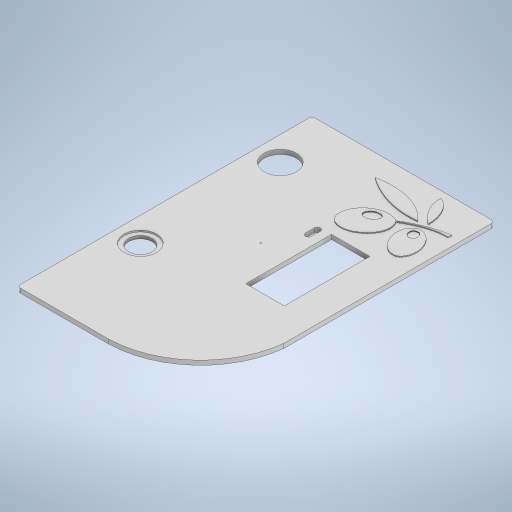
# Autodesk Inventor part: EvoTest_body
Saved by Autodesk Inventor 2023.2 (Build 272271000, 271)
## iProperties
Created: 2022-12-05
Part Number: EvoTest_body
Material: Generico
Document SubType Name: Modeling
Designer: Silvio Marano
Density: 1 g/cm^3
Appearance: Default
Engineer: Silvio Marano
Author: Silvio Marano
Title: EVOTest
Autodesk Inventor part; units mm, degrees
ref_plane "YZ Plane" through (0, 0, 0) normal (1, 0, 0) x (0, 1, 0)
ref_plane "XZ Plane" through (0, 0, 0) normal (0, 1, 0) x (-1, 0, 0)
ref_plane "XY Plane" through (0, 0, 0) normal (0, 0, 1) x (1, 0, 0)
sketch "MainSketch" plane through (0, 0, 0) normal (0, 1, 0) x (-1, 0, 0)
  line L0 (31, -50) -> (-31, -50)
  line L1 (-31, -50) -> (-31, 50)
  line L2 (-31, 50) -> (31, 50)
  line L3 (31, 50) -> (31, -50)
  line L4 (31, -49.4494) -> (-31, 50.5506) construction
  line L5 (-31, -50) -> (31, 50) construction
  line L6 (31, 50) -> (-31, 50)
  line L7 (-31, 50) -> (-31, 21.5)
  line L8 (-31, 21.5) -> (31, 21.5)
  line L9 (31, 21.5) -> (31, 50)
  line L10 (-31, -50) -> (16, -50)
  line L11 (16, -50) -> (16, 21.5)
  line L12 (16, 21.5) -> (-31, 21.5)
  line L13 (-31, 21.5) -> (-31, -50)
  line L14 (31, 21.5) -> (16, 21.5)
  line L15 (16, 21.5) -> (16, -50)
  line L16 (16, -50) -> (31, -50)
  line L17 (31, -50) -> (31, 21.5)
  line L18 (-31, 21.5) -> (-31, 35.75)
  line L19 (-31, 21.5) -> (-31, 35.75)
  arc A0 (0, 50) -> (-31, 21.5) centre (0.8091, 18.0102) ccw
  line L20 (29.5, 48.5) -> (-29.5, 48.5)
  line L21 (-29.5, 48.5) -> (-29.5, -48.5)
  line L22 (-29.5, -48.5) -> (29.5, -48.5)
  line L23 (29.5, -48.5) -> (29.5, 48.5)
  line L24 (29.5, 48.5) -> (-29.5, -48.5) construction
  line L25 (-29.5, 48.5) -> (29.5, -48.5) construction
  line L26 (-29.5, -48.5) -> (16, -48.5)
  line L27 (16, -48.5) -> (16, 2.2597)
  line L28 (16, 2.2597) -> (-29.5, 2.2597)
  line L29 (-29.5, 2.2597) -> (-29.5, -48.5)
  line L30 (16, -48.5) -> (29.5, -48.5)
  line L31 (29.5, -48.5) -> (29.5, 11.5)
  line L32 (29.5, 11.5) -> (16, 11.5)
  line L33 (16, 11.5) -> (16, -48.5)
  line L34 (29.5, 21.5) -> (16, 21.5)
  line L35 (16, 21.5) -> (16, 11.5)
  line L36 (16, 11.5) -> (29.5, 11.5)
  line L37 (29.5, 11.5) -> (29.5, 21.5)
  line L38 (29.5, 21.5) -> (29.5, 11.5)
  line L39 (29.5, 16.5) -> (16, 16.5)
  line L40 (22.75, 16.5) -> (22.75, 11.5)
  line L41 (22.75, 16.5) -> (22.75, 21.5)
  circle A1 centre (22.75, 16.5) radius 4
  arc A2 (0, 48.5) -> (-29.5, 21.5) centre (0.9166, 17.8828) ccw
  line L42 (-20.0675, 15.4609) -> (-7.0675, 15.4609)
  line L43 (-7.0675, 15.4609) -> (-7.0675, -23.5689)
  line L44 (-7.0675, -23.5689) -> (-20.0675, -23.5689)
  line L45 (-20.0675, -23.5689) -> (-20.0675, 15.4609)
  line L46 (22.75, 11.5) -> (22.75, -28.5)
  line L47 (22.75, 11.5) -> (62.75, 11.5) construction
  line L48 (20.2505, -33.5) -> (20.2505, -28.5)
  line L49 (22.75, -28.5) -> (25.2505, -28.5)
  line L50 (20.2505, -28.5) -> (25.2505, -28.5)
  line L51 (25.2505, -28.5) -> (25.2505, -33.5)
  line L52 (25.2505, -33.5) -> (20.2505, -33.5)
  line L53 (20.2505, -33.5) -> (20.2505, -28.5)
  line L54 (25.2505, -28.5) -> (20.2505, -33.5)
  line L55 (20.2505, -28.5) -> (25.2505, -33.5)
  circle A3 centre (22.7505, -31) radius 5.5
  line L56 (-7.0675, 15.4609) -> (-20.0675, 15.4609)
  line L57 (-20.0675, 15.4609) -> (-20.0675, 10.4609)
  line L58 (-20.0675, 10.4609) -> (-7.0675, 10.4609)
  line L59 (-7.0675, 10.4609) -> (-7.0675, 15.4609)
  line L60 (-7.0675, -23.5689) -> (-20.0675, -23.5689)
  line L61 (-20.0675, -23.5689) -> (-20.0675, -18.5689)
  line L62 (-20.0675, -18.5689) -> (-7.0675, -18.5689)
  line L63 (-7.0675, -18.5689) -> (-7.0675, -23.5689)
  line L64 (-29.5, -48.5) -> (-16.5, -48.5)
  line L65 (-16.5, -48.5) -> (-8.5, -48.5)
  line L66 (-8.5, -48.5) -> (-8.5, -42.5)
  line L67 (-8.5, -42.5) -> (-16.5, -42.5)
  line L68 (-16.5, -42.5) -> (-16.5, -48.5)
  line L69 (-8.5, -42.5) -> (-4.5, -42.5)
  line L70 (-8.5, -42.5) -> (-4.5, -42.5) construction
  line L71 (-4.5, -42.5) -> (-3.5, -42.5)
  line L72 (-3.5, -42.5) -> (-3.5, -40.5)
  line L73 (-3.5, -40.5) -> (-4.5, -40.5)
  line L74 (-4.5, -40.5) -> (-4.5, -42.5)
  line L75 (-4.5, -42.5) -> (-3.5, -42.5)
  line L76 (-3.5, -42.5) -> (-3.5, -44.5)
  line L77 (-3.5, -44.5) -> (-4.5, -44.5)
  line L78 (-4.5, -44.5) -> (-4.5, -42.5)
  line L79 (-8.5, -42.5) -> (-8.5, -10.5)
  line L80 (-8.5, -10.5) -> (-10.5, -10.5)
  line L81 (-10.5, -10.5) -> (-10.5, -9.5)
  line L82 (-10.5, -9.5) -> (-8.5, -9.5)
  line L83 (-8.5, -9.5) -> (-8.5, -10.5)
  line L84 (-8.5, -42.5) -> (-8.5, -37.5)
  line L85 (-8.5, -37.5) -> (-9.5, -37.5)
  line L86 (-9.5, -37.5) -> (-9.5, -39.5)
  line L87 (-9.5, -39.5) -> (-8.5, -39.5)
  line L88 (-8.5, -39.5) -> (-8.5, -37.5)
  point P0 (0, 0)
  dimension "d0" = 62
  dimension "d1" = 100
  dimension "d2" = 62
  dimension "d3" = 28.5
  dimension "d4" = 47
  dimension "d5" = 32
  dimension "d6" = 59
  dimension "d7" = 97
  dimension "d8" = 60
  dimension "d9" = 8
  dimension "d10" = 39.0299
  dimension "d11" = 13
  dimension "d12" = 40
  dimension "d13" = 90
  dimension "d14" = 5
  dimension "d15" = 5
  dimension "d16" = 11
  dimension "d17" = 5
  dimension "d18" = 5
  dimension "d19" = 13
  dimension "d20" = 8
  dimension "d21" = 6
  dimension "d22" = 4
  dimension "d23" = 0
  dimension "d24" = 1
  dimension "d25" = 2
  dimension "d26" = 2
  dimension "d27" = 32
  dimension "d28" = 2
  dimension "d29" = 1
  dimension "d30" = 5
  dimension "d31" = 1
  dimension "d32" = 2
  constraints: 178 end point, 32 parallel, 21 perpendicular, 19 horizontal, 12 midpoint, 12 point on line, 4 centre point, 4 point on circle, 2 equal length, 2 vertical, 1 coincident, 1 collinear
  measures "d0" distance of L2.start L2.end
  measures "d1" distance of L3.end L2.end
  measures "d2" distance of L8.end L7.end
  measures "d3" distance of L7.end L6.end
  measures "d4" distance of L12.end L11.end
  measures "d5" radius of A0
  measures "d6" distance of L22.end L21.end
  measures "d7" distance of L21.end L20.end
  measures "d8" distance of L31.end L30.end
  measures "d9" diameter of A1
  measures "d10" distance of L44.end L42.start
  measures "d11" distance of L43.end L44.end
  measures "d12" distance of L40.end L46.end
  measures "d13" angle of L46 L47
  measures "d14" distance of L51.end L48.start
  measures "d15" distance of L49.end L51.end
  measures "d16" diameter of A3
  measures "d17" distance of L57.end L56.end
  measures "d18" distance of L60.end L61.end
  measures "d19" distance of L21.end L64.end
  measures "d20" distance of L67.end L66.end
  measures "d21" distance of L66.end L65.end
  measures "d22" distance of L66.end L69.end
  measures "d23" distance between parallel lines of L69 L70
  measures "d24" distance of L73.end L72.end
  measures "d25" distance of L72.end L71.end
  measures "d26" distance of L75.end L76.end
  measures "d27" distance of L66.end L79.end
  measures "d28" distance of L79.end L80.end
  measures "d29" distance of L80.end L81.end
  measures "d30" distance of L66.end L84.end
  measures "d31" distance of L87.end L86.end
  measures "d32" distance of L86.end L85.end
extrude "MainExtrusion" add sketch "MainSketch" along normal blind 1.5 contours L0 L11 L22 L23 L8 L3 | L0 L1 L8 L21 L22 L11 | L8 L23 L20 A0 L2 L3 | L22 L66 L79 L44 L43 L28 L11 | L11 L32 L23 L22 | L23 L39 A1 L41 L8 | L8 A2 L20 L23 | A0 L21 L8 | L28 L43 L42 L45 L21 L8 L11 | L22 L68 L67 L66 | L41 A1 L39 L11 L8 | L23 L32 L40 A1 L39 | L21 A0 L20 A2 | L11 L39 A1 L40 L32 | L22 L21 L28 L45 L44 L79 L85 L86 L87 L67 L68 | L58 L45 L42 L43 | L43 L44 L79 L62 | L87 L86 L85 L79 | L62 L79 L44 L45 | L74 L73 L72 L71 | L71 L76 L77 L78
sketch "LedSketch" plane through (0, 1.5, 0) normal (0, 1, 0) x (1, 0, 0)
  line L0 (4.2664, 18.5689) -> (2.2664, 18.5689)
  line L1 (2.2664, 18.5689) -> (2.2664, 13.5689)
  line L2 (2.2664, 13.5689) -> (4.2664, 13.5689)
  line L3 (4.2664, 13.5689) -> (4.2664, 18.5689)
  point P0 (0, 0)
  dimension "d35" = 2
  dimension "d36" = 5
  constraints: 8 end point, 2 parallel, 1 horizontal, 1 perpendicular
  measures "d35" distance of L2.end L1.end
  measures "d36" distance of L1.end L0.end
extrude "LedCutExtrusion" cut sketch "LedSketch" against normal blind 1.5
fillet "EdgeConnection" radius 1 3 edges at (-31, 0.75, 50) (-31, 0.75, -50) (31, 0.75, -50)
fillet "LedConnection" radius 1 4 edges at (2.2664, 0.75, -18.5689) (4.2664, 0.75, -18.5689) (4.2664, 0.75, -13.5689) (2.2664, 0.75, -13.5689)
sketch "PipetePlacementSketch" plane through (0, 1.5, 0) normal (0, 1, 0) x (1, 0, 0)
  circle A0 centre (-22.7505, 31) radius 5.5 projected
  line L0 (-17.2505, 31) -> (-17.2505, -16.8177)
  line L1 (-28.2505, 31) -> (-28.2505, -16.8177)
  circle A1 centre (-22.75, -16.5) radius 4 projected
  circle A2 centre (-22.75, -16.5) radius 5.5
  point P0 (0, 0)
  dimension "d41" = 11
  constraints: 4 end point, 2 point on circle, 2 vertical, 1 centre point, 1 coincident, 1 tangent
  measures "d41" diameter of A2
extrude "PipettePlacementExtrusion" cut sketch "PipetePlacementSketch" against normal blind 0.5 contours A2 | A1
sketch "OliveSketch" plane through (0, 1.5, 0) normal (0, 1, 0) x (1, 0, 0)
  line L0 (15.3803, 47.4947) -> (15.7568, 47.3174)
  line L1 (15.7568, 47.3174) -> (16.1189, 47.1219)
  line L2 (16.1189, 47.1219) -> (16.4667, 46.9087)
  line L3 (16.4667, 46.9087) -> (16.8002, 46.6788)
  line L4 (16.8002, 46.6788) -> (17.1196, 46.4328)
  line L5 (17.1196, 46.4328) -> (17.4248, 46.1716)
  line L6 (17.4248, 46.1716) -> (17.716, 45.896)
  line L7 (17.716, 45.896) -> (17.9932, 45.6067)
  line L8 (17.9932, 45.6067) -> (18.2565, 45.3044)
  line L9 (18.2565, 45.3044) -> (18.5059, 44.99)
  line L10 (18.5059, 44.99) -> (18.7416, 44.6642)
  line L11 (18.7416, 44.6642) -> (18.9635, 44.3278)
  line L12 (18.9635, 44.3278) -> (19.1717, 43.9816)
  line L13 (19.1717, 43.9816) -> (19.3664, 43.6263)
  line L14 (19.3664, 43.6263) -> (19.5475, 43.2628)
  line L15 (19.5475, 43.2628) -> (19.7151, 42.8917)
  line L16 (19.7151, 42.8917) -> (19.8694, 42.5139)
  line L17 (19.8694, 42.5139) -> (20.0103, 42.1301)
  line L18 (20.0103, 42.1301) -> (20.138, 41.7412)
  line L19 (20.138, 41.7412) -> (20.2525, 41.3478)
  line L20 (20.2525, 41.3478) -> (20.3538, 40.9508)
  line L21 (20.3538, 40.9508) -> (20.4421, 40.5509)
  line L22 (20.4421, 40.5509) -> (20.5173, 40.1489)
  line L23 (20.5173, 40.1489) -> (20.5796, 39.7455)
  line L24 (20.5796, 39.7455) -> (20.6291, 39.3416)
  line L25 (20.6291, 39.3416) -> (20.6657, 38.938)
  line L26 (20.6657, 38.938) -> (20.6896, 38.5353)
  line L27 (20.6896, 38.5353) -> (20.7009, 38.1344)
  line L28 (20.7009, 38.1344) -> (20.6995, 37.736)
  line L29 (20.6995, 37.736) -> (20.377, 37.9653)
  line L30 (20.377, 37.9653) -> (20.0601, 38.2051)
  line L31 (20.0601, 38.2051) -> (19.7493, 38.4548)
  line L32 (19.7493, 38.4548) -> (19.4452, 38.7144)
  line L33 (19.4452, 38.7144) -> (19.1481, 38.9834)
  line L34 (19.1481, 38.9834) -> (18.8586, 39.2615)
  line L35 (18.8586, 39.2615) -> (18.5771, 39.5486)
  line L36 (18.5771, 39.5486) -> (18.3041, 39.8442)
  line L37 (18.3041, 39.8442) -> (18.04, 40.148)
  line L38 (18.04, 40.148) -> (17.7855, 40.4598)
  line L39 (17.7855, 40.4598) -> (17.5409, 40.7792)
  line L40 (17.5409, 40.7792) -> (17.3067, 41.106)
  line L41 (17.3067, 41.106) -> (17.0833, 41.4399)
  line L42 (17.0833, 41.4399) -> (16.8714, 41.7805)
  line L43 (16.8714, 41.7805) -> (16.6713, 42.1275)
  line L44 (16.6713, 42.1275) -> (16.4835, 42.4807)
  line L45 (16.4835, 42.4807) -> (16.3085, 42.8398)
  line L46 (16.3085, 42.8398) -> (16.1468, 43.2044)
  line L47 (16.1468, 43.2044) -> (15.9988, 43.5742)
  line L48 (15.9988, 43.5742) -> (15.8651, 43.949)
  line L49 (15.8651, 43.949) -> (15.746, 44.3284)
  line L50 (15.746, 44.3284) -> (15.6422, 44.7121)
  line L51 (15.6422, 44.7121) -> (15.554, 45.0999)
  line L52 (15.554, 45.0999) -> (15.4819, 45.4915)
  line L53 (15.4819, 45.4915) -> (15.4265, 45.8865)
  line L54 (15.4265, 45.8865) -> (15.3881, 46.2846)
  line L55 (15.3881, 46.2846) -> (15.3673, 46.6855)
  line L56 (15.3673, 46.6855) -> (15.3646, 47.089)
  line L57 (15.3646, 47.089) -> (15.3803, 47.4947)
  line L58 (-1.9352, 42.3819) -> (-1.212, 42.5249)
  line L59 (-1.212, 42.5249) -> (-0.4813, 42.6475)
  line L60 (-0.4813, 42.6475) -> (0.2559, 42.7493)
  line L61 (0.2559, 42.7493) -> (0.9983, 42.8299)
  line L62 (0.9983, 42.8299) -> (1.7448, 42.889)
  line L63 (1.7448, 42.889) -> (2.4944, 42.9262)
  line L64 (2.4944, 42.9262) -> (3.2458, 42.9412)
  line L65 (3.2458, 42.9412) -> (3.9981, 42.9335)
  line L66 (3.9981, 42.9335) -> (4.75, 42.9028)
  line L67 (4.75, 42.9028) -> (5.5004, 42.8488)
  line L68 (5.5004, 42.8488) -> (6.2482, 42.7711)
  line L69 (6.2482, 42.7711) -> (6.9923, 42.6693)
  line L70 (6.9923, 42.6693) -> (7.7316, 42.543)
  line L71 (7.7316, 42.543) -> (8.4649, 42.3919)
  line L72 (8.4649, 42.3919) -> (9.1912, 42.2157)
  line L73 (9.1912, 42.2157) -> (9.9092, 42.0139)
  line L74 (9.9092, 42.0139) -> (10.6179, 41.7862)
  line L75 (10.6179, 41.7862) -> (11.3162, 41.5323)
  line L76 (11.3162, 41.5323) -> (12.0029, 41.2517)
  line L77 (12.0029, 41.2517) -> (12.6769, 40.9442)
  line L78 (12.6769, 40.9442) -> (13.337, 40.6093)
  line L79 (13.337, 40.6093) -> (13.9823, 40.2466)
  line L80 (13.9823, 40.2466) -> (14.6115, 39.8559)
  line L81 (14.6115, 39.8559) -> (15.2234, 39.4367)
  line L82 (15.2234, 39.4367) -> (15.8171, 38.9888)
  line L83 (15.8171, 38.9888) -> (16.3914, 38.5116)
  line L84 (16.3914, 38.5116) -> (16.9451, 38.0049)
  line L85 (16.9451, 38.0049) -> (17.4771, 37.4683)
  line L86 (17.4771, 37.4683) -> (17.9864, 36.9015)
  line L87 (17.9864, 36.9015) -> (17.2597, 36.8206)
  line L88 (17.2597, 36.8206) -> (16.5319, 36.7617)
  line L89 (16.5319, 36.7617) -> (15.8036, 36.7245)
  line L90 (15.8036, 36.7245) -> (15.0751, 36.7088)
  line L91 (15.0751, 36.7088) -> (14.3468, 36.7142)
  line L92 (14.3468, 36.7142) -> (13.6192, 36.7403)
  line L93 (13.6192, 36.7403) -> (12.8927, 36.787)
  line L94 (12.8927, 36.787) -> (12.1677, 36.8539)
  line L95 (12.1677, 36.8539) -> (11.4447, 36.9407)
  line L96 (11.4447, 36.9407) -> (10.7242, 37.0471)
  line L97 (10.7242, 37.0471) -> (10.0064, 37.1727)
  line L98 (10.0064, 37.1727) -> (9.292, 37.3173)
  line L99 (9.292, 37.3173) -> (8.5812, 37.4806)
  line L100 (8.5812, 37.4806) -> (7.8746, 37.6623)
  line L101 (7.8746, 37.6623) -> (7.1725, 37.862)
  line L102 (7.1725, 37.862) -> (6.4755, 38.0794)
  line L103 (6.4755, 38.0794) -> (5.7838, 38.3143)
  line L104 (5.7838, 38.3143) -> (5.098, 38.5663)
  line L105 (5.098, 38.5663) -> (4.4186, 38.8352)
  line L106 (4.4186, 38.8352) -> (3.7458, 39.1205)
  line L107 (3.7458, 39.1205) -> (3.0802, 39.4221)
  line L108 (3.0802, 39.4221) -> (2.4222, 39.7396)
  line L109 (2.4222, 39.7396) -> (1.7722, 40.0727)
  line L110 (1.7722, 40.0727) -> (1.1306, 40.4211)
  line L111 (1.1306, 40.4211) -> (0.498, 40.7845)
  line L112 (0.498, 40.7845) -> (-0.1254, 41.1626)
  line L113 (-0.1254, 41.1626) -> (-0.739, 41.555)
  line L114 (-0.739, 41.555) -> (-1.3424, 41.9616)
  line L115 (-1.3424, 41.9616) -> (-1.9352, 42.3819)
  line L116 (14.2641, 33.2049) -> (14.7001, 33.4684)
  line L117 (14.7001, 33.4684) -> (15.1391, 33.7274)
  line L118 (15.1391, 33.7274) -> (15.5812, 33.9817)
  line L119 (15.5812, 33.9817) -> (16.0262, 34.2311)
  line L120 (16.0262, 34.2311) -> (16.4741, 34.4756)
  line L121 (16.4741, 34.4756) -> (16.925, 34.7148)
  line L122 (16.925, 34.7148) -> (17.3787, 34.9488)
  line L123 (17.3787, 34.9488) -> (17.8352, 35.1773)
  line L124 (17.8352, 35.1773) -> (18.2944, 35.4002)
  line L125 (18.2944, 35.4002) -> (18.7564, 35.6173)
  line L126 (18.7564, 35.6173) -> (19.221, 35.8285)
  line L127 (19.221, 35.8285) -> (19.6883, 36.0335)
  line L128 (19.6883, 36.0335) -> (20.1582, 36.2324)
  line L129 (20.1582, 36.2324) -> (20.6306, 36.4248)
  line L130 (20.6306, 36.4248) -> (21.1055, 36.6107)
  line L131 (21.1055, 36.6107) -> (21.5829, 36.7898)
  line L132 (21.5829, 36.7898) -> (22.0627, 36.9621)
  line L133 (22.0627, 36.9621) -> (22.5449, 37.1273)
  line L134 (22.5449, 37.1273) -> (23.0294, 37.2854)
  line L135 (23.0294, 37.2854) -> (23.5162, 37.436)
  line L136 (23.5162, 37.436) -> (24.0052, 37.5792)
  line L137 (24.0052, 37.5792) -> (24.4965, 37.7147)
  line L138 (24.4965, 37.7147) -> (24.9899, 37.8424)
  line L139 (24.9899, 37.8424) -> (25.4855, 37.9621)
  line L140 (25.4855, 37.9621) -> (25.9831, 38.0736)
  line L141 (25.9831, 38.0736) -> (26.4828, 38.1769)
  line L142 (26.4828, 38.1769) -> (26.9845, 38.2717)
  line L143 (26.9845, 38.2717) -> (27.4882, 38.3579)
  line L144 (27.4882, 38.3579) -> (27.9937, 38.4353)
  line L145 (27.9937, 38.4353) -> (27.8198, 37.2908)
  line L146 (27.8198, 37.2908) -> (27.3273, 37.294)
  line L147 (27.3273, 37.294) -> (26.8366, 37.2826)
  line L148 (26.8366, 37.2826) -> (26.3475, 37.2569)
  line L149 (26.3475, 37.2569) -> (25.8603, 37.2173)
  line L150 (25.8603, 37.2173) -> (25.375, 37.1643)
  line L151 (25.375, 37.1643) -> (24.8916, 37.0983)
  line L152 (24.8916, 37.0983) -> (24.4103, 37.0197)
  line L153 (24.4103, 37.0197) -> (23.9311, 36.9289)
  line L154 (23.9311, 36.9289) -> (23.4541, 36.8264)
  line L155 (23.4541, 36.8264) -> (22.9794, 36.7127)
  line L156 (22.9794, 36.7127) -> (22.5071, 36.5881)
  line L157 (22.5071, 36.5881) -> (22.0372, 36.453)
  line L158 (22.0372, 36.453) -> (21.5697, 36.3079)
  line L159 (21.5697, 36.3079) -> (21.1049, 36.1533)
  line L160 (21.1049, 36.1533) -> (20.6426, 35.9894)
  line L161 (20.6426, 35.9894) -> (20.1832, 35.8169)
  line L162 (20.1832, 35.8169) -> (19.7265, 35.6361)
  line L163 (19.7265, 35.6361) -> (19.2727, 35.4473)
  line L164 (19.2727, 35.4473) -> (18.8218, 35.2512)
  line L165 (18.8218, 35.2512) -> (18.374, 35.048)
  line L166 (18.374, 35.048) -> (17.9292, 34.8382)
  line L167 (17.9292, 34.8382) -> (17.4877, 34.6223)
  line L168 (17.4877, 34.6223) -> (17.0493, 34.4006)
  line L169 (17.0493, 34.4006) -> (16.6143, 34.1737)
  line L170 (16.6143, 34.1737) -> (16.1828, 33.9418)
  line L171 (16.1828, 33.9418) -> (15.7546, 33.7055)
  line L172 (15.7546, 33.7055) -> (15.3301, 33.4652)
  line L173 (15.3301, 33.4652) -> (14.9091, 33.2212)
  line L174 (14.9091, 33.2212) -> (14.4919, 32.9741)
  line L175 (14.4919, 32.9741) -> (14.7249, 32.6067)
  line L176 (14.7249, 32.6067) -> (14.9206, 32.2342)
  line L177 (14.9206, 32.2342) -> (15.0804, 31.8573)
  line L178 (15.0804, 31.8573) -> (15.2055, 31.4771)
  line L179 (15.2055, 31.4771) -> (15.2972, 31.0942)
  line L180 (15.2972, 31.0942) -> (15.3568, 30.7095)
  line L181 (15.3568, 30.7095) -> (15.3855, 30.3239)
  line L182 (15.3855, 30.3239) -> (15.3846, 29.9381)
  line L183 (15.3846, 29.9381) -> (15.3553, 29.5531)
  line L184 (15.3553, 29.5531) -> (15.299, 29.1696)
  line L185 (15.299, 29.1696) -> (15.2169, 28.7884)
  line L186 (15.2169, 28.7884) -> (15.1103, 28.4104)
  line L187 (15.1103, 28.4104) -> (14.9804, 28.0364)
  line L188 (14.9804, 28.0364) -> (14.8285, 27.6673)
  line L189 (14.8285, 27.6673) -> (14.656, 27.3039)
  line L190 (14.656, 27.3039) -> (14.464, 26.9469)
  line L191 (14.464, 26.9469) -> (14.2538, 26.5973)
  line L192 (14.2538, 26.5973) -> (14.0267, 26.2559)
  line L193 (14.0267, 26.2559) -> (13.784, 25.9234)
  line L194 (13.784, 25.9234) -> (13.5269, 25.6008)
  line L195 (13.5269, 25.6008) -> (13.2567, 25.2888)
  line L196 (13.2567, 25.2888) -> (12.9747, 24.9883)
  line L197 (12.9747, 24.9883) -> (12.6821, 24.7001)
  line L198 (12.6821, 24.7001) -> (12.3803, 24.4251)
  line L199 (12.3803, 24.4251) -> (12.0705, 24.164)
  line L200 (12.0705, 24.164) -> (11.7539, 23.9177)
  line L201 (11.7539, 23.9177) -> (11.4318, 23.687)
  line L202 (11.4318, 23.687) -> (11.1056, 23.4728)
  line L203 (11.1056, 23.4728) -> (10.7764, 23.2759)
  line L204 (10.7764, 23.2759) -> (10.5074, 23.1056)
  line L205 (10.5074, 23.1056) -> (10.2247, 22.9458)
  line L206 (10.2247, 22.9458) -> (9.9297, 22.797)
  line L207 (9.9297, 22.797) -> (9.6237, 22.6599)
  line L208 (9.6237, 22.6599) -> (9.3081, 22.5351)
  line L209 (9.3081, 22.5351) -> (8.9843, 22.4231)
  line L210 (8.9843, 22.4231) -> (8.6537, 22.3245)
  line L211 (8.6537, 22.3245) -> (8.3176, 22.2399)
  line L212 (8.3176, 22.2399) -> (7.9775, 22.1699)
  line L213 (7.9775, 22.1699) -> (7.6347, 22.1151)
  line L214 (7.6347, 22.1151) -> (7.2907, 22.076)
  line L215 (7.2907, 22.076) -> (6.9467, 22.0534)
  line L216 (6.9467, 22.0534) -> (6.6042, 22.0476)
  line L217 (6.6042, 22.0476) -> (6.2645, 22.0594)
  line L218 (6.2645, 22.0594) -> (5.9291, 22.0894)
  line L219 (5.9291, 22.0894) -> (5.5993, 22.138)
  line L220 (5.5993, 22.138) -> (5.2765, 22.2059)
  line L221 (5.2765, 22.2059) -> (4.9621, 22.2937)
  line L222 (4.9621, 22.2937) -> (4.6574, 22.402)
  line L223 (4.6574, 22.402) -> (4.3639, 22.5313)
  line L224 (4.3639, 22.5313) -> (4.0829, 22.6823)
  line L225 (4.0829, 22.6823) -> (3.8158, 22.8555)
  line L226 (3.8158, 22.8555) -> (3.564, 23.0515)
  line L227 (3.564, 23.0515) -> (3.3289, 23.271)
  line L228 (3.3289, 23.271) -> (3.1119, 23.5144)
  line L229 (3.1119, 23.5144) -> (2.9142, 23.7824)
  line L230 (2.9142, 23.7824) -> (2.7374, 24.0756)
  line L231 (2.7374, 24.0756) -> (2.5828, 24.3945)
  line L232 (2.5828, 24.3945) -> (2.4518, 24.7398)
  line L233 (2.4518, 24.7398) -> (2.3711, 25.345)
  line L234 (2.3711, 25.345) -> (2.3498, 25.947)
  line L235 (2.3498, 25.947) -> (2.3852, 26.5437)
  line L236 (2.3852, 26.5437) -> (2.4747, 27.133)
  line L237 (2.4747, 27.133) -> (2.6154, 27.7128)
  line L238 (2.6154, 27.7128) -> (2.8045, 28.281)
  line L239 (2.8045, 28.281) -> (3.0395, 28.8353)
  line L240 (3.0395, 28.8353) -> (3.3175, 29.3737)
  line L241 (3.3175, 29.3737) -> (3.6358, 29.894)
  line L242 (3.6358, 29.894) -> (3.9918, 30.394)
  line L243 (3.9918, 30.394) -> (4.3826, 30.8717)
  line L244 (4.3826, 30.8717) -> (4.8055, 31.3249)
  line L245 (4.8055, 31.3249) -> (5.2578, 31.7514)
  line L246 (5.2578, 31.7514) -> (5.7368, 32.1491)
  line L247 (5.7368, 32.1491) -> (6.2398, 32.5159)
  line L248 (6.2398, 32.5159) -> (6.7639, 32.8496)
  line L249 (6.7639, 32.8496) -> (7.3065, 33.1481)
  line L250 (7.3065, 33.1481) -> (7.8649, 33.4092)
  line L251 (7.8649, 33.4092) -> (8.4362, 33.6309)
  line L252 (8.4362, 33.6309) -> (9.0178, 33.8109)
  line L253 (9.0178, 33.8109) -> (9.607, 33.9471)
  line L254 (9.607, 33.9471) -> (10.201, 34.0375)
  line L255 (10.201, 34.0375) -> (10.7971, 34.0798)
  line L256 (10.7971, 34.0798) -> (11.3925, 34.072)
  line L257 (11.3925, 34.072) -> (11.9845, 34.0118)
  line L258 (11.9845, 34.0118) -> (12.5704, 33.8971)
  line L259 (12.5704, 33.8971) -> (13.1475, 33.7259)
  line L260 (13.1475, 33.7259) -> (13.713, 33.4958)
  line L261 (13.713, 33.4958) -> (14.2641, 33.2049)
  line L262 (8.4112, 32.4895) -> (8.2751, 32.4544)
  line L263 (8.2751, 32.4544) -> (8.1391, 32.4101)
  line L264 (8.1391, 32.4101) -> (8.0036, 32.3573)
  line L265 (8.0036, 32.3573) -> (7.8693, 32.2961)
  line L266 (7.8693, 32.2961) -> (7.7369, 32.2272)
  line L267 (7.7369, 32.2272) -> (7.6068, 32.1508)
  line L268 (7.6068, 32.1508) -> (7.4798, 32.0674)
  line L269 (7.4798, 32.0674) -> (7.3563, 31.9773)
  line L270 (7.3563, 31.9773) -> (7.2371, 31.8811)
  line L271 (7.2371, 31.8811) -> (7.1227, 31.7792)
  line L272 (7.1227, 31.7792) -> (7.0137, 31.6718)
  line L273 (7.0137, 31.6718) -> (6.9108, 31.5595)
  line L274 (6.9108, 31.5595) -> (6.8144, 31.4427)
  line L275 (6.8144, 31.4427) -> (6.7253, 31.3217)
  line L276 (6.7253, 31.3217) -> (6.6441, 31.197)
  line L277 (6.6441, 31.197) -> (6.5712, 31.069)
  line L278 (6.5712, 31.069) -> (6.5074, 30.9381)
  line L279 (6.5074, 30.9381) -> (6.4533, 30.8048)
  line L280 (6.4533, 30.8048) -> (6.4094, 30.6693)
  line L281 (6.4094, 30.6693) -> (6.3763, 30.5323)
  line L282 (6.3763, 30.5323) -> (6.3547, 30.3939)
  line L283 (6.3547, 30.3939) -> (6.3451, 30.2548)
  line L284 (6.3451, 30.2548) -> (6.3482, 30.1152)
  line L285 (6.3482, 30.1152) -> (6.3645, 29.9757)
  line L286 (6.3645, 29.9757) -> (6.3947, 29.8365)
  line L287 (6.3947, 29.8365) -> (6.4394, 29.6982)
  line L288 (6.4394, 29.6982) -> (6.4991, 29.5611)
  line L289 (6.4991, 29.5611) -> (6.5745, 29.4257)
  line L290 (6.5745, 29.4257) -> (6.6661, 29.2923)
  line L291 (6.6661, 29.2923) -> (6.8504, 29.1836)
  line L292 (6.8504, 29.1836) -> (7.0433, 29.0952)
  line L293 (7.0433, 29.0952) -> (7.2436, 29.0262)
  line L294 (7.2436, 29.0262) -> (7.4498, 28.9763)
  line L295 (7.4498, 28.9763) -> (7.6608, 28.9447)
  line L296 (7.6608, 28.9447) -> (7.8752, 28.9308)
  line L297 (7.8752, 28.9308) -> (8.0918, 28.9341)
  line L298 (8.0918, 28.9341) -> (8.3092, 28.9539)
  line L299 (8.3092, 28.9539) -> (8.5261, 28.9897)
  line L300 (8.5261, 28.9897) -> (8.7413, 29.0407)
  line L301 (8.7413, 29.0407) -> (8.9535, 29.1065)
  line L302 (8.9535, 29.1065) -> (9.1614, 29.1864)
  line L303 (9.1614, 29.1864) -> (9.3636, 29.2798)
  line L304 (9.3636, 29.2798) -> (9.5589, 29.3861)
  line L305 (9.5589, 29.3861) -> (9.7461, 29.5047)
  line L306 (9.7461, 29.5047) -> (9.9237, 29.635)
  line L307 (9.9237, 29.635) -> (10.0905, 29.7763)
  line L308 (10.0905, 29.7763) -> (10.2452, 29.9282)
  line L309 (10.2452, 29.9282) -> (10.3866, 30.0899)
  line L310 (10.3866, 30.0899) -> (10.5133, 30.2609)
  line L311 (10.5133, 30.2609) -> (10.624, 30.4405)
  line L312 (10.624, 30.4405) -> (10.7175, 30.6282)
  line L313 (10.7175, 30.6282) -> (10.7924, 30.8233)
  line L314 (10.7924, 30.8233) -> (10.8474, 31.0253)
  line L315 (10.8474, 31.0253) -> (10.8814, 31.2335)
  line L316 (10.8814, 31.2335) -> (10.8929, 31.4473)
  line L317 (10.8929, 31.4473) -> (10.8806, 31.6661)
  line L318 (10.8806, 31.6661) -> (10.8434, 31.8894)
  line L319 (10.8434, 31.8894) -> (10.7798, 32.1165)
  line L320 (10.7798, 32.1165) -> (10.7195, 32.1834)
  line L321 (10.7195, 32.1834) -> (10.656, 32.2445)
  line L322 (10.656, 32.2445) -> (10.5896, 32.3001)
  line L323 (10.5896, 32.3001) -> (10.5204, 32.3504)
  line L324 (10.5204, 32.3504) -> (10.4486, 32.3955)
  line L325 (10.4486, 32.3955) -> (10.3744, 32.4358)
  line L326 (10.3744, 32.4358) -> (10.298, 32.4713)
  line L327 (10.298, 32.4713) -> (10.2195, 32.5023)
  line L328 (10.2195, 32.5023) -> (10.1391, 32.5291)
  line L329 (10.1391, 32.5291) -> (10.057, 32.5518)
  line L330 (10.057, 32.5518) -> (9.8884, 32.5858)
  line L331 (9.8884, 32.5858) -> (9.7152, 32.6061)
  line L332 (9.7152, 32.6061) -> (9.4497, 32.6144)
  line L333 (9.4497, 32.6144) -> (9.0927, 32.593)
  line L334 (9.0927, 32.593) -> (8.4112, 32.4895)
  line L335 (20.5124, 34.6997) -> (21.0739, 34.7213)
  line L336 (21.0739, 34.7213) -> (21.6187, 34.6781)
  line L337 (21.6187, 34.6781) -> (22.1456, 34.5739)
  line L338 (22.1456, 34.5739) -> (22.653, 34.4126)
  line L339 (22.653, 34.4126) -> (23.1394, 34.1979)
  line L340 (23.1394, 34.1979) -> (23.6034, 33.9337)
  line L341 (23.6034, 33.9337) -> (24.0436, 33.6239)
  line L342 (24.0436, 33.6239) -> (24.4585, 33.2723)
  line L343 (24.4585, 33.2723) -> (24.8467, 32.8827)
  line L344 (24.8467, 32.8827) -> (25.2066, 32.459)
  line L345 (25.2066, 32.459) -> (25.537, 32.0049)
  line L346 (25.537, 32.0049) -> (25.8362, 31.5244)
  line L347 (25.8362, 31.5244) -> (26.1028, 31.0212)
  line L348 (26.1028, 31.0212) -> (26.3354, 30.4993)
  line L349 (26.3354, 30.4993) -> (26.5326, 29.9623)
  line L350 (26.5326, 29.9623) -> (26.6929, 29.4143)
  line L351 (26.6929, 29.4143) -> (26.8148, 28.8589)
  line L352 (26.8148, 28.8589) -> (26.8968, 28.3001)
  line L353 (26.8968, 28.3001) -> (26.9378, 27.7416)
  line L354 (26.9378, 27.7416) -> (26.9358, 27.1874)
  line L355 (26.9358, 27.1874) -> (26.8897, 26.6412)
  line L356 (26.8897, 26.6412) -> (26.7979, 26.1069)
  line L357 (26.7979, 26.1069) -> (26.659, 25.5883)
  line L358 (26.659, 25.5883) -> (26.4716, 25.0893)
  line L359 (26.4716, 25.0893) -> (26.2343, 24.6137)
  line L360 (26.2343, 24.6137) -> (25.9454, 24.1653)
  line L361 (25.9454, 24.1653) -> (25.6037, 23.7479)
  line L362 (25.6037, 23.7479) -> (25.2077, 23.3655)
  line L363 (25.2077, 23.3655) -> (24.7558, 23.0218)
  line L364 (24.7558, 23.0218) -> (24.1501, 22.896)
  line L365 (24.1501, 22.896) -> (23.5601, 22.8541)
  line L366 (23.5601, 22.8541) -> (22.9877, 22.8909)
  line L367 (22.9877, 22.8909) -> (22.4348, 23.0013)
  line L368 (22.4348, 23.0013) -> (21.9032, 23.1801)
  line L369 (21.9032, 23.1801) -> (21.3949, 23.4222)
  line L370 (21.3949, 23.4222) -> (20.9118, 23.7226)
  line L371 (20.9118, 23.7226) -> (20.4558, 24.0761)
  line L372 (20.4558, 24.0761) -> (20.0288, 24.4775)
  line L373 (20.0288, 24.4775) -> (19.6327, 24.9218)
  line L374 (19.6327, 24.9218) -> (19.2695, 25.4038)
  line L375 (19.2695, 25.4038) -> (18.9409, 25.9185)
  line L376 (18.9409, 25.9185) -> (18.649, 26.4607)
  line L377 (18.649, 26.4607) -> (18.3955, 27.0253)
  line L378 (18.3955, 27.0253) -> (18.1826, 27.6071)
  line L379 (18.1826, 27.6071) -> (18.0119, 28.2011)
  line L380 (18.0119, 28.2011) -> (17.8855, 28.8021)
  line L381 (17.8855, 28.8021) -> (17.8052, 29.405)
  line L382 (17.8052, 29.405) -> (17.773, 30.0047)
  line L383 (17.773, 30.0047) -> (17.7907, 30.5961)
  line L384 (17.7907, 30.5961) -> (17.8603, 31.1741)
  line L385 (17.8603, 31.1741) -> (17.9837, 31.7335)
  line L386 (17.9837, 31.7335) -> (18.1627, 32.2692)
  line L387 (18.1627, 32.2692) -> (18.3993, 32.7762)
  line L388 (18.3993, 32.7762) -> (18.6953, 33.2492)
  line L389 (18.6953, 33.2492) -> (19.0528, 33.6831)
  line L390 (19.0528, 33.6831) -> (19.4735, 34.073)
  line L391 (19.4735, 34.073) -> (19.9594, 34.4135)
  line L392 (19.9594, 34.4135) -> (20.5124, 34.6997)
  line L393 (20.7048, 33.5997) -> (20.5251, 33.5294)
  line L394 (20.5251, 33.5294) -> (20.3662, 33.4427)
  line L395 (20.3662, 33.4427) -> (20.2275, 33.3412)
  line L396 (20.2275, 33.3412) -> (20.1085, 33.2263)
  line L397 (20.1085, 33.2263) -> (20.0085, 33.0998)
  line L398 (20.0085, 33.0998) -> (19.9271, 32.9631)
  line L399 (19.9271, 32.9631) -> (19.8637, 32.8177)
  line L400 (19.8637, 32.8177) -> (19.8175, 32.6654)
  line L401 (19.8175, 32.6654) -> (19.7882, 32.5076)
  line L402 (19.7882, 32.5076) -> (19.7751, 32.3459)
  line L403 (19.7751, 32.3459) -> (19.7776, 32.1819)
  line L404 (19.7776, 32.1819) -> (19.7952, 32.017)
  line L405 (19.7952, 32.017) -> (19.8272, 31.853)
  line L406 (19.8272, 31.853) -> (19.8731, 31.6914)
  line L407 (19.8731, 31.6914) -> (19.9324, 31.5336)
  line L408 (19.9324, 31.5336) -> (20.0044, 31.3814)
  line L409 (20.0044, 31.3814) -> (20.0886, 31.2362)
  line L410 (20.0886, 31.2362) -> (20.1844, 31.0996)
  line L411 (20.1844, 31.0996) -> (20.2912, 30.9732)
  line L412 (20.2912, 30.9732) -> (20.4085, 30.8585)
  line L413 (20.4085, 30.8585) -> (20.5356, 30.7571)
  line L414 (20.5356, 30.7571) -> (20.6721, 30.6707)
  line L415 (20.6721, 30.6707) -> (20.8172, 30.6006)
  line L416 (20.8172, 30.6006) -> (20.9705, 30.5485)
  line L417 (20.9705, 30.5485) -> (21.1313, 30.5161)
  line L418 (21.1313, 30.5161) -> (21.2992, 30.5047)
  line L419 (21.2992, 30.5047) -> (21.4734, 30.516)
  line L420 (21.4734, 30.516) -> (21.6535, 30.5516)
  line L421 (21.6535, 30.5516) -> (21.8389, 30.613)
  line L422 (21.8389, 30.613) -> (22.0205, 30.6814)
  line L423 (22.0205, 30.6814) -> (22.1816, 30.7671)
  line L424 (22.1816, 30.7671) -> (22.3227, 30.8686)
  line L425 (22.3227, 30.8686) -> (22.4442, 30.9842)
  line L426 (22.4442, 30.9842) -> (22.5468, 31.1121)
  line L427 (22.5468, 31.1121) -> (22.631, 31.2508)
  line L428 (22.631, 31.2508) -> (22.6973, 31.3986)
  line L429 (22.6973, 31.3986) -> (22.7462, 31.5539)
  line L430 (22.7462, 31.5539) -> (22.7783, 31.7149)
  line L431 (22.7783, 31.7149) -> (22.7941, 31.8801)
  line L432 (22.7941, 31.8801) -> (22.7941, 32.0478)
  line L433 (22.7941, 32.0478) -> (22.7789, 32.2163)
  line L434 (22.7789, 32.2163) -> (22.749, 32.3839)
  line L435 (22.749, 32.3839) -> (22.7048, 32.549)
  line L436 (22.7048, 32.549) -> (22.6471, 32.71)
  line L437 (22.6471, 32.71) -> (22.5762, 32.8652)
  line L438 (22.5762, 32.8652) -> (22.4928, 33.0128)
  line L439 (22.4928, 33.0128) -> (22.3973, 33.1514)
  line L440 (22.3973, 33.1514) -> (22.2903, 33.2792)
  line L441 (22.2903, 33.2792) -> (22.1724, 33.3945)
  line L442 (22.1724, 33.3945) -> (22.044, 33.4958)
  line L443 (22.044, 33.4958) -> (21.9057, 33.5813)
  line L444 (21.9057, 33.5813) -> (21.758, 33.6494)
  line L445 (21.758, 33.6494) -> (21.6015, 33.6985)
  line L446 (21.6015, 33.6985) -> (21.4367, 33.7268)
  line L447 (21.4367, 33.7268) -> (21.264, 33.7327)
  line L448 (21.264, 33.7327) -> (21.0842, 33.7146)
  line L449 (21.0842, 33.7146) -> (20.8976, 33.6709)
  line L450 (20.8976, 33.6709) -> (20.7048, 33.5997)
  point P0 (0, 0)
  constraints: 902 end point, 10 parallel, 5 perpendicular
emboss "OliveEmbossment" sketch "OliveSketch" operation add depth 0.3 direction (0, -1, 0)
